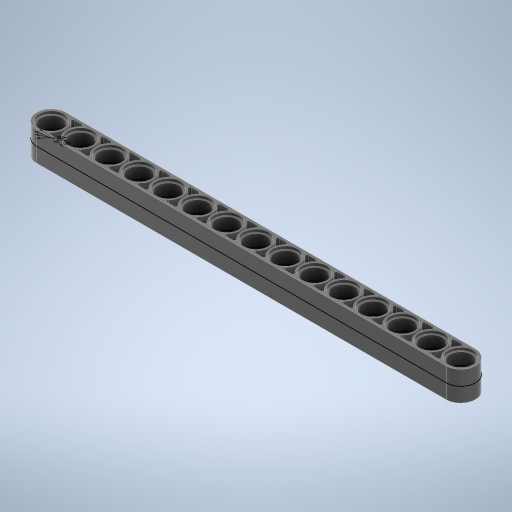
# Autodesk Inventor part: Beam1x15
Saved by Autodesk Inventor 2024.1 (Build 281209000, 209)
## iProperties
Created: 2023-11-23
Part Number: Beam1x15
Material: Generic
Document SubType Name: Modeling
Designer: njona
Density: 1 g/cm^3
Appearance: Smooth - Black
Author: njona
Autodesk Inventor part; units mm, degrees
ref_plane "YZ Plane" through (0, 0, 0) normal (1, 0, 0) x (0, 1, 0)
ref_plane "XZ Plane" through (0, 0, 0) normal (0, 1, 0) x (-1, 0, 0)
ref_plane "XY Plane" through (0, 0, 0) normal (0, 0, 1) x (1, 0, 0)
sketch "Sketch1" plane through (0, 0, 0) normal (0, 1, 0) x (-1, 0, 0)
  circle A0 centre (177.8, 0) radius 12.065
  circle A1 centre (177.8, 0) radius 10.795
  circle A2 centre (177.8, 0) radius 12.7
  circle A3 centre (177.8, 0) radius 9.525
  circle A4 centre (152.4, 0) radius 12.065
  circle A5 centre (152.4, 0) radius 10.795
  circle A6 centre (152.4, 0) radius 12.7 construction
  circle A7 centre (152.4, 0) radius 9.525
  circle A8 centre (127, 0) radius 12.065
  circle A9 centre (127, 0) radius 10.795
  circle A10 centre (127, 0) radius 12.7 construction
  circle A11 centre (127, 0) radius 9.525
  circle A12 centre (101.6, 0) radius 12.065
  circle A13 centre (101.6, 0) radius 10.795
  circle A14 centre (101.6, 0) radius 12.7 construction
  circle A15 centre (101.6, 0) radius 9.525
  circle A16 centre (76.2, 0) radius 12.065
  circle A17 centre (76.2, 0) radius 10.795
  circle A18 centre (76.2, 0) radius 12.7 construction
  circle A19 centre (76.2, 0) radius 9.525
  circle A20 centre (50.8, 0) radius 12.065
  circle A21 centre (50.8, 0) radius 10.795
  circle A22 centre (50.8, 0) radius 12.7 construction
  circle A23 centre (50.8, 0) radius 9.525
  circle A24 centre (25.4, 0) radius 9.525
  circle A25 centre (25.4, 0) radius 10.795
  circle A26 centre (25.4, 0) radius 12.065
  circle A27 centre (25.4, 0) radius 12.7 construction
  circle A28 centre (0, 0) radius 9.525
  circle A29 centre (0, 0) radius 10.795
  circle A30 centre (0, 0) radius 12.065
  circle A31 centre (0, 0) radius 12.7 construction
  circle A32 centre (-25.4, 0) radius 9.525
  circle A33 centre (-25.4, 0) radius 10.795
  circle A34 centre (-25.4, 0) radius 12.065
  circle A35 centre (-25.4, 0) radius 12.7 construction
  circle A36 centre (-50.8, 0) radius 9.525
  circle A37 centre (-50.8, 0) radius 10.795
  circle A38 centre (-50.8, 0) radius 12.065
  circle A39 centre (-50.8, 0) radius 12.7 construction
  circle A40 centre (-76.2, 0) radius 12.065
  circle A41 centre (-76.2, 0) radius 10.795
  circle A42 centre (-76.2, 0) radius 12.7 construction
  circle A43 centre (-76.2, 0) radius 9.525
  circle A44 centre (-101.6, 0) radius 9.525
  circle A45 centre (-101.6, 0) radius 10.795
  circle A46 centre (-101.6, 0) radius 12.065
  circle A47 centre (-101.6, 0) radius 12.7 construction
  circle A48 centre (-127, 0) radius 9.525
  circle A49 centre (-127, 0) radius 10.795
  circle A50 centre (-127, 0) radius 12.065
  circle A51 centre (-127, 0) radius 12.7 construction
  circle A52 centre (-152.4, 0) radius 9.525
  circle A53 centre (-152.4, 0) radius 10.795
  circle A54 centre (-152.4, 0) radius 12.065
  circle A55 centre (-152.4, 0) radius 12.7 construction
  circle A56 centre (-177.8, 0) radius 9.525
  circle A57 centre (-177.8, 0) radius 10.795
  circle A58 centre (-177.8, 0) radius 12.065
  circle A59 centre (-177.8, 0) radius 12.7
  line L0 (177.8, -12.7) -> (-177.8, -12.7)
  line L1 (177.8, -12.065) -> (-177.8, -12.065)
  line L2 (177.8, -10.795) -> (-177.8, -10.795)
  line L3 (-177.8, -9.525) -> (177.8, -9.525) construction
  line L4 (177.8, 12.7) -> (-177.8, 12.7)
  line L5 (177.8, 12.065) -> (-177.8, 12.065)
  line L6 (177.8, 10.795) -> (-177.8, 10.795)
  point P0 (132.3882, 10.795)
  point P1 (147.0118, 10.795)
  point P2 (147.0118, -10.795)
  point P3 (132.3882, -10.795)
  point P4 (157.7882, 10.795)
  point P5 (172.4118, 10.795)
  point P6 (172.4118, -10.795)
  point P7 (157.7882, -10.795)
  point P8 (127, 12.065)
  point P9 (121.6118, -10.795)
  point P10 (106.9882, -10.795)
  point P11 (101.6, -12.065)
  point P12 (-172.4118, 10.795)
  point P13 (-157.7882, 10.795)
  point P14 (-157.7882, -10.795)
  point P15 (-172.4118, -10.795)
  point P16 (-147.0118, 10.795)
  point P17 (-132.3882, 10.795)
  point P18 (-132.3882, -10.795)
  point P19 (-147.0118, -10.795)
  point P20 (-121.6118, 10.795)
  point P21 (-106.9882, 10.795)
  point P22 (-106.9882, -10.795)
  point P23 (-121.6118, -10.795)
  point P24 (-96.2118, 10.795)
  point P25 (-81.5882, 10.795)
  point P26 (-81.5882, -10.795)
  point P27 (-96.2118, -10.795)
  point P28 (-70.8118, 10.795)
  point P29 (-56.1882, 10.795)
  point P30 (-56.1882, -10.795)
  point P31 (-70.8118, -10.795)
  point P32 (-45.4118, 10.795)
  point P33 (-30.7882, 10.795)
  point P34 (-30.7882, -10.795)
  point P35 (-45.4118, -10.795)
  point P36 (-20.0118, 10.795)
  point P37 (-5.3882, 10.795)
  point P38 (-5.3882, -10.795)
  point P39 (-20.0118, -10.795)
  point P40 (5.3882, 10.795)
  point P41 (20.0118, 10.795)
  point P42 (20.0118, -10.795)
  point P43 (5.3882, -10.795)
  point P44 (30.7882, 10.795)
  point P45 (45.4118, 10.795)
  point P46 (45.4118, -10.795)
  point P47 (30.7882, -10.795)
  point P48 (56.1882, 10.795)
  point P49 (70.8118, 10.795)
  point P50 (70.8118, -10.795)
  point P51 (56.1882, -10.795)
  point P52 (81.5882, 10.795)
  point P53 (96.2118, 10.795)
  point P54 (96.2118, -10.795)
  point P55 (81.5882, -10.795)
  point P56 (106.9882, 10.795)
  point P57 (121.6118, 10.795)
  dimension "d31" = 19.05
  dimension "d32" = 21.59
  dimension "d33" = 24.13
  dimension "d34" = 25.4
  constraints: 60 tangent, 58 centre point, 46 coincident, 14 equal radius, 12 point on circle, 10 end point, 5 horizontal, 2 parallel, 2 vertical alignment, 27 other
  measures "d32" diameter of A1
  measures "d33" diameter of A0
  measures "d34" diameter of A2
extrude "Extrusion9" add sketch "Sketch1" along normal mid plane 25.4 contours A0 L2 A1 L6 | A0 L5 A2 L1 | A0 L6 A2 L5 | L1 A2 L2 A0 | L6 A1 L2 A0 | L5 A59 L4 A2 | A2 L6 A4 L5 | L1 A4 L2 A2 | A2 L0 A59 L1 | A4 L6 | A4 L6 A8 L5 | L1 A8 L2 A4 | A4 L2 | A4 L2 A5 L6 | A59 L5 A58 L1 | L6 A5 L2 A4 | A8 L6 | A8 L6 A12 L5 | L1 A12 L2 A8 | A8 L2 | L5 A54 L6 A59 | A59 L6 A58 L5 | A8 L2 A9 L6 | L6 A9 L2 A8 | A12 L6 | A12 L6 A16 L5 | L1 A58 L2 A59 | A59 L2 A54 L1 | L1 A16 L2 A12 | A12 L2 | L5 A50 L6 A54 | A54 L6 | A58 L6 A57 L2 | A12 L2 A13 L6 | L6 A13 L2 A12 | A16 L6 | A16 L6 A20 L5 | A54 L2 | A54 L2 A50 L1 | L1 A20 L2 A16 | A16 L2 | L6 A53 L2 A54 | A58 L2 A57 L6 | A54 L2 A53 L6 | L5 A46 L6 A50 | A50 L6 | A16 L2 A17 L6 | L6 A17 L2 A16 | A20 L6 | A20 L6 A26 L5 | A50 L2 | A50 L2 A46 L1 | L1 A26 L2 A20 | A20 L2 | L6 A49 L2 A50 | A50 L2 A49 L6 | L5 A40 L6 A46 | A46 L6 | A20 L2 A21 L6 | L6 A21 L2 A20 | A26 L6 | A26 L6 A30 L5 | A46 L2 | A46 L2 A40 L1 | L1 A30 L2 A26 | A26 L2 | L6 A45 L2 A46 | A46 L2 A45 L6 | L5 A38 L6 A40 | A40 L6 | A26 L2 A25 L6 | L6 A25 L2 A26 | A30 L6 | A30 L6 A34 L5 | A40 L2 | A40 L2 A38 L1 | L1 A34 L2 A30 | A30 L2 | L6 A41 L2 A40 | A40 L2 A41 L6 | L5 A34 L6 A38 | A38 L6 | A30 L2 A29 L6 | L6 A29 L2 A30 | A34 L6 | A38 L2 | A38 L2 A34 L1 | A34 L2 | L6 A37 L2 A38 | A38 L2 A37 L6 | A34 L2 A33 L6 | L6 A33 L2 A34
extrude "Extrusion10" add sketch "Sketch1" along normal mid plane 20.32 contours A1 | A5 | A9 | A13 | A53 | A57 | A17 | A49 | A21 | A45 | A25 | A41 | A29 | A37 | A33
extrude "Extrusion11" add sketch "Sketch1" along normal mid plane 3.81 contours A0 L2 A2 L6 | A2 L2 A4 L6 | A4 L2 A8 L6 | A8 L2 A12 L6 | L6 A54 L2 A59 | A59 L2 A58 L6 | A12 L2 A16 L6 | L6 A50 L2 A54 | A16 L2 A20 L6 | L6 A46 L2 A50 | A20 L2 A26 L6 | L6 A40 L2 A46 | A26 L2 A30 L6 | L6 A38 L2 A40 | A30 L2 A34 L6 | L6 A34 L2 A38
fillet "Fillet1" radius 1.27 55 edges at (172.4118, 7.3025, 10.795) (157.7882, 7.3025, 10.795) (172.4118, 7.3025, -10.795) (157.7882, 7.3025, -10.795) (147.0118, 7.3025, -10.795) (147.0118, 7.3025, 10.795) (121.6118, 7.3025, 10.795) (96.2118, 7.3025, 10.795) (70.8118, 7.3025, 10.795) (45.4118, 7.3025, 10.795) (20.0118, 7.3025, 10.795) (-5.3882, 7.3025, 10.795) (-30.7882, 7.3025, 10.795) (-56.1882, 7.3025, 10.795) (-81.5882, 7.3025, 10.795) (-106.9882, 7.3025, 10.795) (-132.3882, 7.3025, 10.795) (-157.7882, 7.3025, 10.795) (-172.4118, 7.3025, 10.795) (-147.0118, 7.3025, 10.795) (-121.6118, 7.3025, 10.795) (-96.2118, 7.3025, 10.795) (-70.8118, 7.3025, 10.795) (-45.4118, 7.3025, 10.795) (-20.0118, 7.3025, 10.795) (5.3882, 7.3025, 10.795) (30.7882, 7.3025, 10.795) (56.1882, 7.3025, 10.795) (81.5882, 7.3025, 10.795) (106.9882, 7.3025, 10.795) (132.3882, 7.3025, 10.795) (121.6118, 7.3025, -10.795) (96.2118, 7.3025, -10.795) (70.8118, 7.3025, -10.795) (45.4118, 7.3025, -10.795) (20.0118, 7.3025, -10.795) (-5.3882, 7.3025, -10.795) (-30.7882, 7.3025, -10.795) (-56.1882, 7.3025, -10.795) (-81.5882, 7.3025, -10.795) (-106.9882, 7.3025, -10.795) (-132.3882, 7.3025, -10.795) (-157.7882, 7.3025, -10.795) (-172.4118, 7.3025, -10.795) (-147.0118, 7.3025, -10.795) (-96.2118, 7.3025, -10.795) (-70.8118, 7.3025, -10.795) (-45.4118, 7.3025, -10.795) (-20.0118, 7.3025, -10.795) (5.3882, 7.3025, -10.795) (30.7882, 7.3025, -10.795) (56.1882, 7.3025, -10.795) (81.5882, 7.3025, -10.795) (106.9882, 7.3025, -10.795) (132.3882, 7.3025, -10.795)
body "Solid4"
